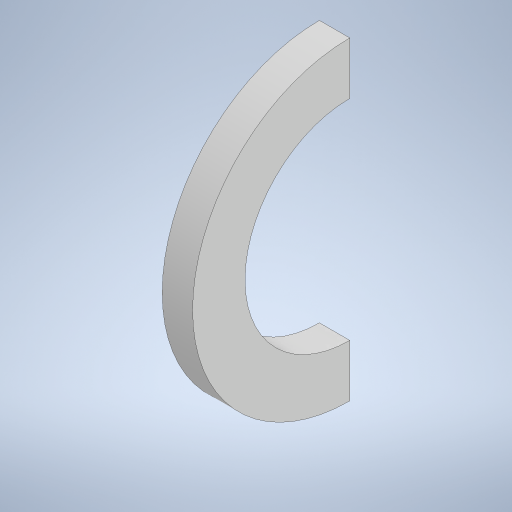
# Autodesk Inventor part: disk_support
Saved by Autodesk Inventor 2023 (Build 270158000, 158)
## iProperties
Created: 2026-05-06
Part Number: disk_support
Material: Generic
Document SubType Name: Modeling
Designer: Justin Pascual
Density: 1 g/cm^3
Appearance: Default
Author: Justin Pascual
Autodesk Inventor part; units mm, degrees
ref_plane "YZ Plane" through (0, 0, 0) normal (1, 0, 0) x (0, 1, 0)
ref_plane "XZ Plane" through (0, 0, 0) normal (0, 1, 0) x (-1, 0, 0)
ref_plane "XY Plane" through (0, 0, 0) normal (0, 0, 1) x (1, 0, 0)
sketch "Sketch1" plane through (0, 0, 0) normal (1, 0, 0) x (0, 1, 0)
  arc A0 (19.05, 0) -> (-19.05, 0) centre (0, 0) ccw
  arc A1 (12.7, 0) -> (-12.7, 0) centre (0, 0) ccw
  line L0 (19.05, 0) -> (-19.05, 0)
  arc A2 (-19.05, 0) -> (19.05, 0) centre (0, 0) ccw construction
  arc A3 (-12.7, 0) -> (12.7, 0) centre (0, 0) ccw construction
  dimension "d0" = 38.1
  dimension "d1" = 25.4
  constraints: 8 point on circle, 4 centre point, 2 coincident, 2 end point, 2 point on line, 1 horizontal
  measures "d0" diameter of A0
  measures "d1" diameter of A1
extrude "Extrusion1" add sketch "Sketch1" along normal blind 3.683 contours L0 A1 A0
body "Solid1"
